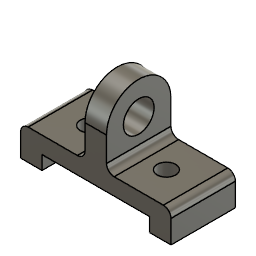
d3 (Autodesk Fusion 360 design; units mm, degrees)
part number: 2026-08-20-18-20-11-075
Autodesk Fusion 360 part; units mm, degrees
sketch "Sketch1" plane through (0, 0, 0) normal (0, 1, 0) x (1, 0, 0)
  line L0 (49, 21) -> (-49, 21)
  line L1 (-49, 21) -> (-49, -21)
  line L2 (-49, -21) -> (49, -21)
  line L3 (49, -21) -> (49, 21)
  line L4 (49, 21) -> (-49, -21) construction
  line L5 (-49, 21) -> (49, -21) construction
  circle A0 centre (25, 0) radius 6
  circle A1 centre (-25, 0) radius 6
  dimension "d1" = 98
  dimension "d2" = 42
  dimension "d3" = 12
  dimension "d4" = 12
  dimension "d5" = 24
  dimension "d6" = 21
  dimension "d8" = 21
  dimension "d16" = 50
  constraint horizontal L0
  constraint perpendicular L0 L1
  constraint parallel L0 L2
  constraint parallel L1 L3
  constraint coincident L4 origin
  constraint coincident L5 origin
  measures "d1" distance of L1.end L2.end
  measures "d2" distance of L0.end L1.end
  measures "d3" diameter of A0
  measures "d4" diameter of A1
  measures "d5" distance of L3 A0.centre
  measures "d6" distance of L2 A0.centre
  measures "d8" distance of L2 A1.centre
  measures "d16" distance of A0.centre A1.centre
extrude "Extrude1" add sketch "Sketch1" along normal blind 20
sketch "Sketch2" plane through (0, 0, 21) normal (0, 0, 1) x (1, 0, 0)
  line L0 (-49, 0) -> (49, 0)
  line L1 (49, 0) -> (49, 20)
  line L2 (49, 20) -> (-49, 20)
  line L3 (-49, 20) -> (-49, 0)
  line L4 (-35, 0) -> (35, 0)
  line L5 (35, 0) -> (35, 9)
  line L6 (35, 9) -> (-35, 9)
  line L7 (-35, 9) -> (-35, 0)
  dimension "d11" = 70
  dimension "d12" = 9
  dimension "d13" = 14
  constraint horizontal L4
  constraint vertical L5
  constraint horizontal L6
  constraint vertical L7
  constraint coincident L0 L4.start
  measures "d11" distance of L4.start L4.end
  measures "d12" distance of L4.start L6.end
  measures "d13" distance of L0.start L4.start
extrude "Extrude2" cut sketch "Sketch2" against normal blind 42 contours L0 L4 L5 L6 L7
sketch "Sketch3" plane through (0, 20, 0) normal (0, 1, 0) x (-1, 0, 0)
  circle A0 centre (25, 0) radius 6
  circle A1 centre (-25, 0) radius 6
  line L0 (-49, 21) -> (-49, -21)
  line L1 (-49, -21) -> (49, -21)
  line L2 (49, -21) -> (49, 21)
  line L3 (49, 21) -> (-49, 21)
  line L4 (-7, -21) -> (7, -21)
  line L5 (7, -21) -> (7, 21)
  line L6 (7, 21) -> (-7, 21)
  line L7 (-7, 21) -> (-7, -21)
  line L8 (-7, -21) -> (7, 21) construction
  line L9 (7, -21) -> (-7, 21) construction
  dimension "d17" = 14
  dimension "d18" = 42
  constraint horizontal L4
  constraint perpendicular L4 L5
  constraint parallel L4 L6
  constraint parallel L5 L7
  constraint coincident L8 origin
  constraint coincident L9 origin
  measures "d17" distance of L5.end L6.end
  measures "d18" distance of L4.end L5.end
extrude "Extrude3" add sketch "Sketch3" along normal blind 42 contours L1 L3 L4 L5 L6 L7
sketch "Sketch4" plane through (7, 0, 0) normal (1, 0, 0) x (0, 0, -1)
  line L0 (-21, 20) -> (21, 20)
  line L1 (21, 20) -> (21, 62)
  line L2 (21, 62) -> (-21, 62)
  line L3 (-21, 62) -> (-21, 20)
  circle A0 centre (0, 41) radius 10
  arc A1 (21, 41) -> (-21, 41) centre (0, 41) ccw
  dimension "d21" = 42
  dimension "d22" = 21
  constraint concentric A0 A1
  constraint coincident L3 A1.end
  constraint coincident L1 A1.start
  measures "d21" diameter of A1
  measures "d22" distance of L0 A0.centre
extrude "Extrude4" cut sketch "Sketch4" against normal blind 14 contours L2 L3 A1 | L1 L2 A1 | A0
fillet "Fillet1" radius 5 2 edges at (49, 20, 0) (-49, 20, 0)
fillet "Fillet2" radius 5 2 edges at (7, 20, 0) (-7, 20, 0)
